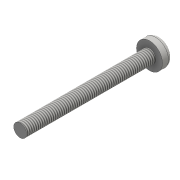
# Autodesk Inventor part: m3 30mm screw
Saved by Autodesk Inventor 2016 (Build 200138000, 138)
## iProperties
Created: 2015-07-05
Part Number: m3 30mm screw
Material: Generic
Document SubType Name: Modeling
Designer: Sebastian
Density: 1 g/cm^3
Appearance: Default
Mass: 0.273322 g
Surface Area: 3.88396 cm^2
Volume: 0.273322 cm^3
Author: Sebastian
Autodesk Inventor part; units mm, degrees
ref_plane "YZ Plane" through (0, 0, 0) normal (1, 0, 0) x (0, 1, 0)
ref_plane "XZ Plane" through (0, 0, 0) normal (0, 1, 0) x (-1, 0, 0)
ref_plane "XY Plane" through (0, 0, 0) normal (0, 0, 1) x (1, 0, 0)
sketch "Sketch1" plane through (0, 0, 0) normal (0, 1, 0) x (-1, 0, 0)
  circle A0 centre (0, 0) radius 3
  dimension "d0" = 6
  constraints: 1 centre point, 1 coincident
  measures "d0" diameter of A0
extrude "Extrusion1" add sketch "Sketch1" along normal blind 2.4
sketch "Sketch2" plane through (0, 2.4, 0) normal (0, 1, 0) x (1, 0, 0)
  line L0 (-1.55, 0.25) -> (1.55, 0.25)
  line L1 (1.55, 0.25) -> (1.55, -0.25)
  line L2 (1.55, -0.25) -> (-1.55, -0.25)
  line L3 (-1.55, -0.25) -> (-1.55, 0.25)
  line L4 (-0.25, -1.55) -> (0.25, -1.55)
  line L5 (0.25, -1.55) -> (0.25, 1.55)
  line L6 (0.25, 1.55) -> (-0.25, 1.55)
  line L7 (-0.25, 1.55) -> (-0.25, -1.55)
  point P0 (0, 0)
  dimension "d5" = 3.1
  dimension "d6" = 0.5
  dimension "d9" = 0.5
  dimension "d10" = 3.1
  constraints: 16 end point, 4 parallel, 2 horizontal, 2 perpendicular
  measures "d5" distance of L1.end L2.end
  measures "d6" distance of L0.end L1.end
  measures "d9" distance of L6.end L5.end
  measures "d10" distance of L5.end L4.end
extrude "Extrusion2" cut sketch "Sketch2" against normal blind 1
fillet "Fillet1" radius 1 1 edges at (3, 2.4, 0)
sketch "Sketch3" plane through (0, 0, 0) normal (0, -1, 0) x (1, 0, 0)
  circle A0 centre (0, 0) radius 1.5
  dimension "d14" = 3
  constraints: 1 centre point, 1 coincident
  measures "d14" diameter of A0
extrude "Extrusion3" add sketch "Sketch3" along normal blind 30
thread "Thread1" size "M3x0.5" class "6g" standard "ANSI Metric M Profile" full length
body "Solid1"
